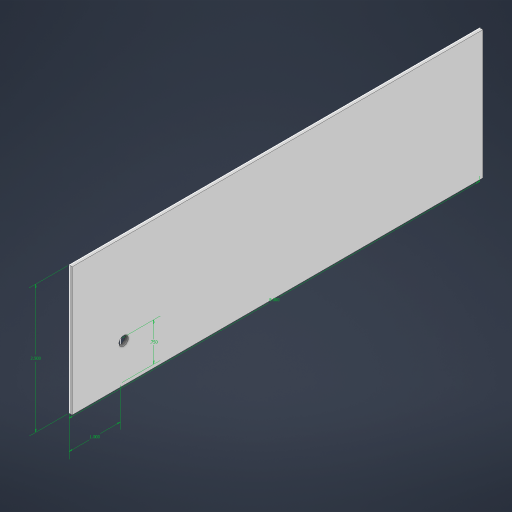
# Autodesk Inventor part: dtplate
Saved by Autodesk Inventor 2024 (Build 280153000, 153)
## iProperties
Created: 2023-11-04
Part Number: dtplate
Material: Generic
Document SubType Name: Modeling
Designer: macbook
Density: 1 g/cm^3
Appearance: Default
Author: macbook
Autodesk Inventor part; units mm, degrees
ref_plane "YZ Plane" through (0, 0, 0) normal (1, 0, 0) x (0, 1, 0)
ref_plane "XZ Plane" through (0, 0, 0) normal (0, 1, 0) x (-1, 0, 0)
ref_plane "XY Plane" through (0, 0, 0) normal (0, 0, 1) x (1, 0, 0)
sketch "Sketch1" plane through (0, 0, 0) normal (1, 0, 0) x (0, 1, 0)
  line L0 (0, 0) -> (0, -203.2)
  line L1 (0, 0) -> (63.5, 0)
  line L2 (0, -203.2) -> (63.5, -203.2)
  line L3 (63.5, -203.2) -> (63.5, 0)
  line L4 (0, 0) -> (0, -25.4)
  line L5 (0, -25.4) -> (19.05, -25.4)
  dimension "d0" = 203.2
  dimension "d1" = 63.5
  dimension "d2" = 25.4
  dimension "d3" = 19.05
  constraints: 12 end point, 2 horizontal, 2 perpendicular, 1 coincident, 1 point on line, 1 vertical
  measures "d0" distance of L0.start L0.end
  measures "d1" distance of L0.start L1.end
  measures "d2" distance of L0.start L4.end
  measures "d3" distance of L4.end L5.end
extrude "Extrusion1" add sketch "Sketch1" along normal blind 1.5875
hole "Hole1" at (0, 19.05, -25.4) direction (1, 0, 0) diameter 4.7625 end through all
body "Solid1"
